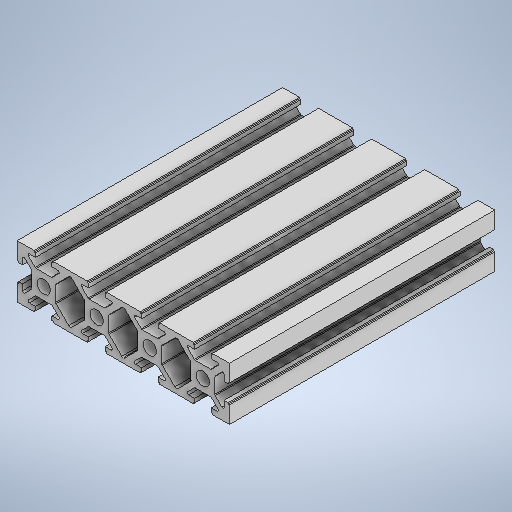
# Autodesk Inventor part: Perfil 20×80 10 rasgos_001
Saved by Autodesk Inventor 2026 (Build 300175000, 175)
## iProperties
Created: 2025-04-02
Part Number: Perfil 20×80 10 rasgos_001
Material: Generic
Document SubType Name: Modeling
Designer: Carlos Dias
Density: 1 g/cm^3
Appearance: Default
Author: Carlos Dias
Autodesk Inventor part; units mm, degrees
sketch "Sketch1" plane through (0, 0, 0) normal (0, 0, 1) x (1, 0, 0)
  line L0 (0, 10) -> (0, 0) construction
  line L1 (-10, 10) -> (0, 10) construction
  circle A0 centre (-10, 0) radius 2.5 construction
  line L2 (10, 20) -> (-10, 0) construction
  line L3 (-14.5, 4.5) -> (-5.5, 4.5) construction
  line L4 (-5.5, 4.5) -> (-5.5, 0) construction
  line L5 (-14.5, 4.5) -> (-14.5, 0) construction
  line L6 (-3.4142, 8) -> (-6.9142, 4.5) construction
  line L7 (-0.5858, 8) -> (-5.5, 3.0858) construction
  line L8 (-6.9, 8) -> (-3.4142, 8) construction
  line L9 (-6.9, 10) -> (-6.9, 8) construction
  line L10 (-19, 9) -> (-10, 0) construction
  line L11 (-16.5858, 8) -> (-13.0858, 4.5) construction
  line L12 (-40, 20) -> (0, 20) construction
  line L13 (-30, 15) -> (0, 15) construction
  line L14 (0, 20) -> (0, 0) construction
  line L15 (-16.5858, 8) -> (-13.1, 8) construction
  line L16 (-19.4142, 8) -> (-14.5, 3.0858) construction
  line L17 (-13.1, 10) -> (-13.1, 8) construction
  circle A1 centre (-30, 0) radius 2.5 construction
  line L18 (-34.5, 4.5) -> (-25.5, 4.5) construction
  line L19 (-25.5, 4.5) -> (-25.5, 0) construction
  line L20 (-34.5, 4.5) -> (-34.5, 0) construction
  line L21 (-21, 9) -> (-30, 0) construction
  line L22 (-20.5858, 8) -> (-25.5, 3.0858) construction
  line L23 (-23.4142, 8) -> (-26.9142, 4.5) construction
  line L24 (-26.9, 8) -> (-23.4142, 8) construction
  line L25 (-26.9, 10) -> (-26.9, 8) construction
  line L26 (-39, 9) -> (-30, 0) construction
  line L27 (-36.5858, 8) -> (-33.0858, 4.5) construction
  line L28 (-38, 6.5858) -> (-34.5, 3.0858) construction
  line L29 (-40, 20) -> (-40, 0) construction
  line L30 (-36.5858, 8) -> (-33.1, 8) construction
  line L31 (-33.1, 10) -> (-33.1, 8) construction
  line L32 (-38, 3.1) -> (-38, 6.5858) construction
  line L33 (-38, 3.1) -> (-40, 3.1) construction
  arc A2 (-19.4142, 8) -> (-20.5858, 8) centre (-20, 7.4142) ccw
  arc A3 (-27.5, 0) -> (-32.5, 0) centre (-30, 0) ccw
  arc A4 (-34.5, 2.8787) -> (-34.6464, 3.2322) centre (-35, 2.8787) ccw
  line L34 (-34.5, 2.8787) -> (-34.5, 0)
  line L35 (-34.5, 0) -> (-32.5, 0)
  line L36 (-37.1464, 5.7322) -> (-34.6464, 3.2322)
  arc A5 (-37.1464, 5.7322) -> (-38, 5.3787) centre (-37.5, 5.3787) ccw
  line L37 (-38, 5.3787) -> (-38, 3.1)
  line L38 (-40, 3.1) -> (-39.5, 3.1) construction
  line L39 (-39.5, 3.1) -> (-39.5, 3.6)
  line L40 (-39.5, 3.6) -> (-40, 3.6)
  line L41 (-40, 3.6) -> (-40, 3.1) construction
  line L42 (-39.5, 3.1) -> (-38, 3.1)
  line L43 (-40, 10) -> (-40, 3.6)
  line L44 (-33.1, 10) -> (-33.6, 10) construction
  line L45 (-33.6, 10) -> (-33.6, 9.5)
  line L46 (-33.6, 9.5) -> (-33.1, 9.5)
  line L47 (-33.1, 9.5) -> (-33.1, 10) construction
  line L48 (-33.6, 10) -> (-40, 10)
  line L49 (-33.1, 9.5) -> (-33.1, 8)
  arc A6 (-35.3787, 8) -> (-35.7322, 7.1464) centre (-35.3787, 7.5) ccw
  line L50 (-33.1, 8) -> (-35.3787, 8)
  arc A7 (-33.2322, 4.6464) -> (-32.8787, 4.5) centre (-32.8787, 5) ccw
  line L51 (-35.7322, 7.1464) -> (-33.2322, 4.6464)
  arc A8 (-27.1213, 4.5) -> (-26.7678, 4.6464) centre (-27.1213, 5) ccw
  line L52 (-32.8787, 4.5) -> (-27.1213, 4.5)
  arc A9 (-24.2678, 7.1464) -> (-24.6213, 8) centre (-24.6213, 7.5) ccw
  line L53 (-24.2678, 7.1464) -> (-26.7678, 4.6464)
  line L54 (-24.6213, 8) -> (-26.9, 8)
  line L55 (-26.9, 10) -> (-26.4, 10) construction
  line L56 (-26.4, 10) -> (-26.4, 9.5)
  line L57 (-26.4, 9.5) -> (-26.9, 9.5)
  line L58 (-26.9, 9.5) -> (-26.9, 10) construction
  line L59 (-26.9, 9.5) -> (-26.9, 8)
  line L60 (-13.1, 10) -> (-13.6, 10) construction
  line L61 (-13.6, 10) -> (-13.6, 9.5)
  line L62 (-13.6, 9.5) -> (-13.1, 9.5)
  line L63 (-13.1, 9.5) -> (-13.1, 10) construction
  line L64 (-13.6, 10) -> (-26.4, 10)
  line L65 (-13.1, 9.5) -> (-13.1, 8)
  arc A10 (-15.3787, 8) -> (-15.7322, 7.1464) centre (-15.3787, 7.5) ccw
  line L66 (-13.1, 8) -> (-15.3787, 8)
  line L67 (-20.5858, 8) -> (-25.3536, 3.2322)
  arc A11 (-25.3536, 3.2322) -> (-25.5, 2.8787) centre (-25, 2.8787) ccw
  line L68 (-25.5, 2.8787) -> (-25.5, 0)
  line L69 (-25.5, 0) -> (-27.5, 0)
  arc A12 (-14.5, 2.8787) -> (-14.6464, 3.2322) centre (-15, 2.8787) ccw
  line L70 (-19.4142, 8) -> (-14.6464, 3.2322)
  line L71 (-14.5, 2.8787) -> (-14.5, 0)
  line L72 (-14.5, 0) -> (-12.5, 0)
  arc A13 (-7.5, 0) -> (-12.5, 0) centre (-10, 0) ccw
  arc A14 (-13.2322, 4.6464) -> (-12.8787, 4.5) centre (-12.8787, 5) ccw
  line L73 (-15.7322, 7.1464) -> (-13.2322, 4.6464)
  arc A15 (-7.1213, 4.5) -> (-6.7678, 4.6464) centre (-7.1213, 5) ccw
  line L74 (-12.8787, 4.5) -> (-7.1213, 4.5)
  arc A16 (-4.2678, 7.1464) -> (-4.6213, 8) centre (-4.6213, 7.5) ccw
  line L75 (-4.2678, 7.1464) -> (-6.7678, 4.6464)
  line L76 (-6.9, 8) -> (-4.6213, 8)
  line L77 (-6.9, 10) -> (-6.4, 10) construction
  line L78 (-6.4, 10) -> (-6.4, 9.5)
  line L79 (-6.4, 9.5) -> (-6.9, 9.5)
  line L80 (-6.9, 9.5) -> (-6.9, 10) construction
  line L81 (-6.9, 9.5) -> (-6.9, 8)
  line L82 (-6.4, 10) -> (0, 10)
  arc A17 (0, 8.2341) -> (-0.5858, 8) centre (-0.0201, 7.4343) ccw
  line L83 (0, 10) -> (0, 8.2341)
  arc A18 (-5.3536, 3.2322) -> (-5.5, 2.8787) centre (-5, 2.8787) ccw
  line L84 (-0.5858, 8) -> (-5.3536, 3.2322)
  line L85 (-5.5, 2.8787) -> (-5.5, 0)
  line L86 (-5.5, 0) -> (-7.5, 0)
  point P0 (-30, 4.5)
  dimension "d2" = 5
  dimension "d0" = 10
  dimension "d1" = 10
  dimension "d3" = 4.5
  dimension "d4" = 4.5
  dimension "d5" = 1
  dimension "d6" = 2
  dimension "d7" = 1
  dimension "d8" = 3.1
  dimension "d10" = 1
  dimension "d11" = 40
  dimension "d12" = 30
  dimension "d13" = 20
  dimension "d14" = 15
  dimension "d17" = 1
  dimension "d19" = 1
  dimension "d20" = 1
  dimension "d22" = 1
  dimension "d23" = 1
  dimension "d24" = 2
  dimension "d28" = 0.5
  dimension "d29" = 0.5
  dimension "d30" = 0.5
  dimension "d31" = 0.5
  dimension "d32" = 0.5
  dimension "d33" = 0.5
  dimension "d34" = 0.5
  dimension "d35" = 0.5
  dimension "d36" = 0.5
  dimension "d37" = 0.5
  dimension "d38" = 0.5
  dimension "d39" = 0.5
  dimension "d40" = 0.5
  dimension "d41" = 0.8
  dimension "d42" = 0.5
  constraints: 174 end point, 38 point on line, 34 point on circle, 29 horizontal, 28 tangent, 21 equal length, 21 vertical, 20 horizontal alignment, 18 centre point, 18 parallel, 7 midpoint, 5 perpendicular, 5 vertical alignment, 3 coincident, 2 concentric, 5 other
  measures "d0" distance of L0.start L0.end
  measures "d1" distance of L0.start L1.start
  measures "d3" distance from line of point (-10, 0) L3
  measures "d4" distance from line of L5 point (-10, 0)
  measures "d5" distance between parallel lines of L2 L6
  measures "d6" distance from line of L1 L6.start
  measures "d7" distance between parallel lines of L2 L7
  measures "d8" horizontal distance of point (-10, 0) L8.start
  measures "d10" distance between parallel lines of L10 L11
  measures "d11" distance of L12.start L12.end
  measures "d12" distance of L13.start L13.end
  measures "d13" distance of point (0, 0) L12.end
  measures "d14" distance of point (0, 0) L13.end
  measures "d17" distance between parallel lines of L10 L16
  measures "d19" distance between parallel lines of L21 L22
  measures "d20" distance between parallel lines of L21 L23
  measures "d22" distance between parallel lines of L26 L27
  measures "d23" distance between parallel lines of L26 L28
  measures "d24" distance from line of L29 L28.start
  measures "d28" radius of A4
  measures "d29" radius of A5
  measures "d30" distance of L39.end L40.end
  measures "d31" radius of A6
  measures "d32" radius of A7
  measures "d33" radius of A8
  measures "d34" radius of A9
  measures "d35" radius of A10
  measures "d36" radius of A11
  measures "d37" radius of A12
  measures "d38" radius of A14
  measures "d39" radius of A15
  measures "d40" radius of A16
  measures "d41" radius of A17
  measures "d42" radius of A18
extrude "Extrusion1" add sketch "Sketch1" along normal mid plane 100
mirror "Mirror1" about plane through (0, 0, 0) normal (0, 1, 0) of "Extrusion1"
mirror "Mirror2" about plane through (0, 0, 0) normal (1, 0, 0) of "Extrusion1", "Mirror1"
equation "\"d4\" = d3"
equation "\"d7\" = d5"
equation "\"d10\" = d5"
equation "\"d17\" = d5"
equation "\"d19\" = d5"
equation "\"d20\" = d5"
equation "\"d22\" = d5"
equation "\"d23\" = d5"
equation "\"d29\" = d28"
equation "\"d31\" = d28"
equation "\"d32\" = d28"
equation "\"d33\" = d28"
body "Solid1"
